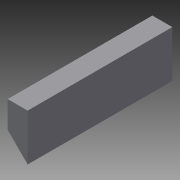
# Autodesk Inventor part: ShieldMount2x4
Saved by Autodesk Inventor 2014 (Build 180170000, 170)
## iProperties
Created: 2016-02-03
Part Number: ShieldMount2x4
Material: Generic
Document SubType Name: Modeling
Designer: zoldberg
Density: 1 g/cm^3
Appearance: Default
Author: zoldberg
Autodesk Inventor part; units mm, degrees
ref_plane "YZ Plane" through (0, 0, 0) normal (1, 0, 0) x (0, 1, 0)
ref_plane "XZ Plane" through (0, 0, 0) normal (0, 1, 0) x (-1, 0, 0)
ref_plane "XY Plane" through (0, 0, 0) normal (0, 0, 1) x (1, 0, 0)
sketch "Sketch1" plane through (0, 0, 0) normal (0, 0, 1) x (1, 0, 0)
  line L0 (-19.05, -44.45) -> (19.05, -44.45)
  line L1 (19.05, -44.45) -> (19.05, 44.45)
  line L2 (19.05, 44.45) -> (-19.05, 44.45)
  line L3 (-19.05, 44.45) -> (-19.05, -44.45)
  line L4 (-19.05, -44.45) -> (19.05, 44.45) construction
  line L5 (19.05, -44.45) -> (-19.05, 44.45) construction
  point P0 (0, 0)
  dimension "d0" = 38.1
  dimension "d1" = 88.9
  constraints: 12 end point, 2 midpoint, 2 parallel, 1 horizontal, 1 perpendicular
  measures "d0" distance of L2.end L1.end
  measures "d1" distance of L1.end L0.end
extrude "Extrusion1" add sketch "Sketch1" along normal blind 275.8186
chamfer "Chamfer1" distance 38.1 angle 45 1 edges at (-19.05, -44.45, 137.9093)
body "Solid1"
